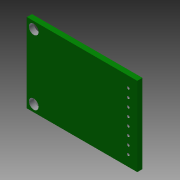
# Autodesk Inventor part: arducam'
Saved by Autodesk Inventor 2015 SP1 (Build 190203100, 203)
## iProperties
Created: 2015-10-23
Part Number: arducam'
Material: Generic
Document SubType Name: Modeling
Designer: Kartikye
Density: 1 g/cm^3
Appearance: Default
Author: Kartikye
Autodesk Inventor part; units mm, degrees
ref_plane "YZ Plane" through (0, 0, 0) normal (1, 0, 0) x (0, 1, 0)
ref_plane "XZ Plane" through (0, 0, 0) normal (0, 1, 0) x (-1, 0, 0)
ref_plane "XY Plane" through (0, 0, 0) normal (0, 0, 1) x (1, 0, 0)
sketch "Sketch1" plane through (0, 0, 0) normal (0, 1, 0) x (-1, 0, 0)
  line L0 (-17.05, 12.2) -> (17.05, 12.2)
  line L1 (17.05, 12.2) -> (17.05, -12.2)
  line L2 (17.05, -12.2) -> (-17.05, -12.2)
  line L3 (-17.05, -12.2) -> (-17.05, 12.2)
  line L4 (-17.05, 12.2) -> (17.05, -12.2) construction
  line L5 (17.05, 12.2) -> (-17.05, -12.2) construction
  point P0 (0, 0)
  dimension "d0" = 34.1
  dimension "d1" = 24.4
  constraints: 12 end point, 2 midpoint, 2 parallel, 1 horizontal, 1 perpendicular
  measures "d0" distance of L1.end L2.end
  measures "d1" distance of L0.end L1.end
extrude "Extrusion1" add sketch "Sketch1" along normal blind 1.6
sketch "Sketch2" plane through (0, 1.6, 0) normal (0, 1, 0) x (1, 0, 0)
  circle A0 centre (-14.92, -10) radius 1.5
  circle A1 centre (-14.92, 10) radius 1.5
  line L0 (-17.05, 12.2) -> (-17.05, -12.2) projected
  line L1 (-17.05, -12.2) -> (17.05, -12.2) projected
  line L2 (17.05, 12.2) -> (-17.05, 12.2) projected
  circle A2 centre (14.26, -6.35) radius 0.4
  circle A3 centre (14.26, -3.81) radius 0.4
  circle A4 centre (14.26, -1.27) radius 0.4
  circle A5 centre (14.26, -8.89) radius 0.4
  circle A6 centre (14.26, 1.27) radius 0.4
  line L3 (17.05, -12.2) -> (17.05, 12.2) projected
  circle A7 centre (14.26, 3.81) radius 0.4
  circle A8 centre (14.26, 6.35) radius 0.4
  circle A9 centre (14.26, 8.89) radius 0.4
  point P0 (0, 0)
  dimension "d4" = 3
  dimension "d5" = 3
  dimension "d6" = 2.13
  dimension "d7" = 2.2
  dimension "d8" = 2.13
  dimension "d9" = 2.2
  dimension "d10" = 0.8
  dimension "d11" = 0.8
  dimension "d12" = 2.54
  dimension "d13" = 0.8
  dimension "d14" = 0.8
  dimension "d15" = 0.8
  dimension "d16" = 2.79
  dimension "d17" = 2.54
  dimension "d18" = 2.79
  dimension "d19" = 2.79
  dimension "d20" = 2.79
  dimension "d21" = 2.54
  dimension "d22" = 2.79
  dimension "d23" = 2.54
  dimension "d24" = 0.8
  dimension "d25" = 0.8
  dimension "d26" = 0.8
  dimension "d27" = 2.79
  dimension "d28" = 2.79
  dimension "d29" = 2.79
  dimension "d30" = 2.54
  dimension "d31" = 2.54
  dimension "d32" = 2.54
  dimension "d33" = 3.31
  constraints: 10 centre point
  measures "d4" diameter of A0
  measures "d5" diameter of A1
  measures "d6" distance from line of A0.centre L0
  measures "d7" distance from line of A0.centre L1
  measures "d8" distance from line of A1.centre L0
  measures "d9" distance from line of L2 A1.centre
  measures "d10" diameter of A2
  measures "d11" diameter of A3
  measures "d12" distance of A3.centre A2.centre
  measures "d13" diameter of A4
  measures "d14" diameter of A5
  measures "d15" diameter of A6
  measures "d16" distance from line of A5.centre L3
  measures "d17" distance of A5.centre A2.centre
  measures "d18" distance from line of L3 A2.centre
  measures "d19" distance from line of A3.centre L3
  measures "d20" distance from line of A4.centre L3
  measures "d21" distance of A3.centre A4.centre
  measures "d22" distance from line of L3 A6.centre
  measures "d23" distance of A6.centre A4.centre
  measures "d24" diameter of A7
  measures "d25" diameter of A8
  measures "d26" diameter of A9
  measures "d27" distance from line of A7.centre L3
  measures "d28" distance from line of A8.centre L3
  measures "d29" distance from line of A9.centre L3
  measures "d30" distance of A7.centre A6.centre
  measures "d31" distance of A7.centre A8.centre
  measures "d32" distance of A9.centre A8.centre
  measures "d33" distance from line of L1 A5.centre
extrude "Extrusion2" cut sketch "Sketch2" against normal blind 3.31 contours A0 | A1 | A2 | A3 | A4 | A5 | A6 | A7 | A8 | A9
sketch "Sketch3" plane through (0, 1.6, 0) normal (0, 1, 0) x (1, 0, 0)
  line L0 (-16.05, -7.5) -> (-1.05, -7.5)
  line L1 (-1.05, -7.5) -> (-1.05, 7.5)
  line L2 (-1.05, 7.5) -> (-16.05, 7.5)
  line L3 (-16.05, 7.5) -> (-16.05, -7.5)
  line L4 (-16.05, -7.5) -> (-1.05, 7.5) construction
  line L5 (-1.05, -7.5) -> (-16.05, 7.5) construction
  line L6 (-17.05, 12.2) -> (-17.05, -12.2) projected
  point P0 (0, 0)
  point P1 (-8.55, 0)
  dimension "d36" = 15
  dimension "d37" = 15
  dimension "d38" = 1
  constraints: 12 end point, 2 midpoint, 2 parallel, 1 horizontal, 1 perpendicular
  measures "d36" distance of L2.end L1.end
  measures "d37" distance of L1.end L0.end
  measures "d38" distance between parallel lines of L3 L6
extrude "Extrusion3" add sketch "Sketch3" along normal blind 3.3
equation "\"d34\" = d33"
body "Solid1"
